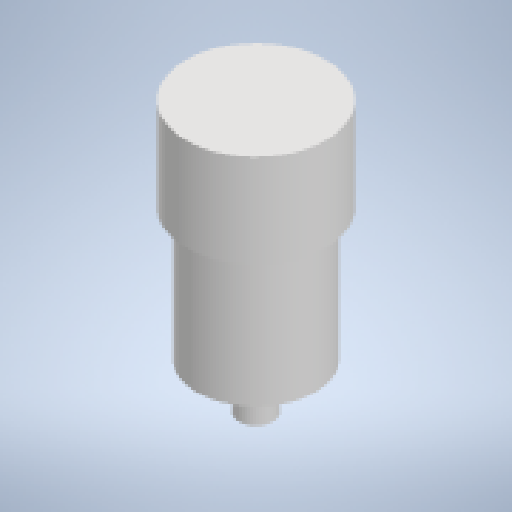
# Autodesk Inventor part: Spindle
Saved by Autodesk Inventor 2023 (Build 270158000, 158)
## iProperties
Created: 2022-05-05
Part Number: Spindle
Material: Generic
Document SubType Name: Modeling
Designer: plebbb
Density: 3.82137 g/cm^3
Appearance: Default
Mass: 3628.74 g
Surface Area: 564.979 cm^2
Volume: 949.592 cm^3
Author: plebbb
Autodesk Inventor part; units mm, degrees
ref_plane "YZ Plane" through (0, 0, 0) normal (1, 0, 0) x (0, 1, 0)
ref_plane "XZ Plane" through (0, 0, 0) normal (0, 1, 0) x (-1, 0, 0)
ref_plane "XY Plane" through (0, 0, 0) normal (0, 0, 1) x (1, 0, 0)
sketch "Sketch1" plane through (0, 0, 0) normal (0, 0, 1) x (1, 0, 0)
  line L0 (0, 0) -> (44.45, 0)
  line L1 (44.45, 0) -> (44.45, 98)
  line L2 (44.45, 98) -> (0, 98)
  line L3 (0, 98) -> (0, 0)
  line L4 (4.7625, 0) -> (0, 0)
  line L5 (0, 0) -> (0, -35)
  line L6 (0, -35) -> (4.7625, -35)
  line L7 (4.7625, -35) -> (4.7625, 0)
  line L8 (4.7625, -35) -> (12.7, -35)
  line L9 (12.7, -35) -> (12.7, 0)
  line L10 (12.7, 0) -> (4.7625, 0)
  line L11 (4.7625, 0) -> (4.7625, -35)
  line L12 (0, 98) -> (52.5, 98)
  line L13 (52.5, 98) -> (52.5, 168)
  line L14 (52.5, 168) -> (0, 168)
  line L15 (0, 168) -> (0, 98)
  dimension "d0" = 44.45
  dimension "d1" = 98
  dimension "d3" = 4.7625
  dimension "d4" = 35
  dimension "d5" = 12.7
  dimension "d6" = 52.5
  dimension "d7" = 70
  constraints: 32 end point, 8 parallel, 4 horizontal, 4 perpendicular, 2 point on line
  measures "d0" distance of L1.end L2.end
  measures "d1" distance of L0.end L1.end
  measures "d3" distance of L5.end L6.end
  measures "d4" distance of L6.end L4.start
  measures "d5" distance of L5.end L8.end
  measures "d6" distance of L13.end L14.end
  measures "d7" distance of L12.end L13.end
revolve "Revolution1" add sketch "Sketch1" angle 360 about axis through (0, 98, 0) along (0, -1, 0) contours L3 L2 L1 L0 | L0 L9 L8 L7 | L15 L14 L13 L12 L2
body "Solid1"
